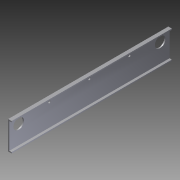
# Autodesk Inventor part: uptake bearing plate
Saved by Autodesk Inventor 2012 (Build 160160000, 160)
## iProperties
Created: 2013-07-07
Part Number: uptake bearing plate
Material: Default
Document SubType Name: Modeling
Designer: Bryce
Density: 1 g/cm^3
Author: Bryce
Autodesk Inventor part; units mm, degrees
ref_plane "YZ Plane" through (0, 0, 0) normal (1, 0, 0) x (0, 1, 0)
ref_plane "XZ Plane" through (0, 0, 0) normal (0, 1, 0) x (-1, 0, 0)
ref_plane "XY Plane" through (0, 0, 0) normal (0, 0, 1) x (1, 0, 0)
sketch "Sketch1" plane through (0, 0, 0) normal (0, 0, 1) x (1, 0, 0)
  line L0 (0, 0) -> (9.525, 0)
  line L1 (9.525, 76.2) -> (0, 76.2)
  line L2 (0, 76.2) -> (0, 0)
  line L3 (9.525, 3.175) -> (3.175, 3.175)
  line L4 (3.175, 3.175) -> (3.175, 73.025)
  line L5 (3.175, 73.025) -> (9.525, 73.025)
  line L6 (9.525, 0) -> (9.525, 3.175)
  line L7 (9.525, 73.025) -> (9.525, 76.2)
  dimension "d0" = 3.175
  dimension "d2" = 3.175
  dimension "d3" = 3.175
  dimension "d4" = 76.2
  dimension "d5" = 9.525
  constraints: 16 end point, 4 parallel, 3 perpendicular, 2 horizontal, 1 vertical alignment
  measures "d0" distance between parallel lines of L1 L5
  measures "d2" distance between parallel lines of L2 L4
  measures "d3" distance between parallel lines of L3 L0
  measures "d4" distance of L1.end L0.start
  measures "d5" distance of L0.start L0.end
extrude "Extrusion1" add sketch "Sketch1" along normal blind 434.975
sketch "Sketch2" plane through (3.175, 3.175, 0) normal (1, 0, 0) x (0, 0, -1)
  line L0 (0, 0) -> (0, 69.85) projected
  line L1 (0, 73.025) -> (-434.975, 73.025) projected
  line L2 (0, -3.175) -> (-434.975, -3.175) projected
  line L3 (-434.975, 0) -> (-434.975, -3.175) projected
  line L4 (-434.975, 73.025) -> (-434.975, 69.85) projected
  line L5 (0, 69.85) -> (0, 73.025) projected
  line L6 (0, -3.175) -> (0, 0) projected
  circle A0 centre (-25.4, 50.8) radius 14.2875
  line L7 (-434.975, 69.85) -> (-434.975, 0) projected
  circle A1 centre (-409.575, 50.8) radius 14.2875
  circle A2 centre (-217.4875, 60.325) radius 3.175
  circle A3 centre (-326.2313, 60.325) radius 3.175
  circle A4 centre (-108.7438, 60.325) radius 3.175
  dimension "d8" = 28.575
  dimension "d10" = 53.975
  dimension "d11" = 25.4
  dimension "d14" = 25.4
  dimension "d15" = 53.975
  dimension "d16" = 28.575
  dimension "d17" = 6.35
  dimension "d18" = 12.7
  dimension "d19" = 217.4875
  dimension "d20" = 108.7438
  dimension "d21" = 108.7438
  dimension "d22" = 6.35
  dimension "d23" = 6.35
  dimension "d24" = 434.975
  constraints: 5 centre point, 2 horizontal alignment
  measures "d8" diameter of A0
  measures "d10" distance from line of L2 A0.centre
  measures "d11" distance from line of L0 A0.centre
  measures "d14" distance from line of L7 A1.centre
  measures "d15" distance from line of L2 A1.centre
  measures "d16" diameter of A1
  measures "d17" diameter of A2
  measures "d18" distance from line of L1 A2.centre
  measures "d19" distance from line of L7 A2.centre
  measures "d20" distance from line of L0 A4.centre
  measures "d21" distance from line of L7 A3.centre
  measures "d22" diameter of A3
  measures "d23" diameter of A4
  measures "d24" distance between parallel lines of L0 L7
extrude "Extrusion2" cut sketch "Sketch2" against normal blind 508 contours A0 | A1 | A2 | A3 | A4
equation "\"d3\" = d2"
equation "\"d14\" = d11"
equation "\"d15\" = d10"
equation "\"d16\" = d8"
equation "\"d19\" = 0.5 * d24"
equation "\"d20\" = d21"
equation "\"d21\" = 0.5 * d19"
equation "\"d22\" = d17"
equation "\"d23\" = d17"
body "Solid1"
